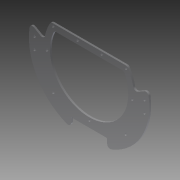
# Autodesk Inventor part: Light Sensor Plate
Saved by Autodesk Inventor 2015 (Build 190159000, 159)
## iProperties
Created: 2016-02-18
Part Number: Light Sensor Plate
Material: Polycarbonate, Clear
Document SubType Name: Modeling
Designer: 23902
Density: 1.2 g/cm^3
Appearance: Polycarbonate - Clear
Mass: 38.1211 g
Surface Area: 243.455 cm^2
Volume: 31.7676 cm^3
Author: 23902
Autodesk Inventor part; units mm, degrees
ref_plane "YZ Plane" through (0, 0, 0) normal (1, 0, 0) x (0, 1, 0)
ref_plane "XZ Plane" through (0, 0, 0) normal (0, 1, 0) x (-1, 0, 0)
ref_plane "XY Plane" through (0, 0, 0) normal (0, 0, 1) x (1, 0, 0)
sketch "Sketch1" plane through (0, 0, 0) normal (0, 1, 0) x (-1, 0, 0)
  circle A0 centre (60.6719, 34.9243) radius 1.6
  circle A1 centre (-60.5717, 34.9243) radius 1.6
  circle A2 centre (0.0501, -70.0757) radius 1.6
  line L0 (-54.4935, 29.9243) -> (54.5936, 29.9243)
  arc A3 (-59.0388, 27.0076) -> (59.1389, 27.0076) centre (0.0501, -0.0757) ccw
  arc A4 (-54.4935, 29.9243) -> (-59.0388, 27.0076) centre (-54.4935, 24.9243) ccw
  arc A5 (59.1389, 27.0076) -> (54.5936, 29.9243) centre (54.5936, 24.9243) ccw
  line L1 (-29.9499, 39.9243) -> (-60.5717, 39.9243)
  line L2 (-29.9499, 39.9243) -> (60.6719, 39.9243)
  arc A6 (-60.5717, 39.9243) -> (-64.9018, 37.4243) centre (-60.5717, 34.9243) ccw
  arc A7 (65.002, 37.4243) -> (60.6719, 39.9243) centre (60.6719, 34.9243) ccw
  line L3 (0.0501, -80.0757) -> (-15.7999, -80.0757)
  line L4 (0.0501, -80.0757) -> (-27.9499, -80.0757)
  arc A8 (-27.9499, -80.0757) -> (-29.9499, -82.0757) centre (-27.9499, -82.0757) ccw
  line L5 (-29.9499, -82.0757) -> (-29.9499, -88.3933)
  arc A9 (-44.5914, -89.5583) -> (-36.792, -93.0416) centre (0.0501, -0.0757) ccw
  arc A10 (-36.792, -93.0416) -> (-29.9499, -88.3933) centre (-34.9499, -88.3933) ccw
  line L6 (0.0501, -80.0757) -> (15.9001, -80.0757)
  line L7 (0.0501, -80.0757) -> (28.0501, -80.0757)
  arc A11 (30.0501, -82.0757) -> (28.0501, -80.0757) centre (28.0501, -82.0757) ccw
  line L8 (30.0501, -82.0757) -> (30.0501, -88.3933)
  arc A12 (36.8922, -93.0416) -> (44.6916, -89.5583) centre (0.0501, -0.0757) ccw
  arc A13 (30.0501, -88.3933) -> (36.8922, -93.0416) centre (35.0501, -88.3933) ccw
  arc A14 (44.6916, -89.5583) -> (98.982, 14.501) centre (0.0501, -0.0757) ccw
  arc A15 (-98.8818, 14.501) -> (-44.5914, -89.5583) centre (0.0501, -0.0757) ccw
  arc A16 (-91.4352, 18.1023) -> (-98.8818, 14.501) centre (-93.9352, 13.7722) ccw
  line L9 (-91.4352, 18.1023) -> (-80.7621, 11.9402)
  arc A17 (-64.9018, 37.4243) -> (-73.3676, 15.2487) centre (0.0501, -0.0757) ccw
  arc A18 (-80.7621, 11.9402) -> (-73.3676, 15.2487) centre (-78.2621, 16.2704) ccw
  arc A19 (98.982, 14.501) -> (91.5354, 18.1023) centre (94.0354, 13.7722) ccw
  line L10 (91.5354, 18.1023) -> (80.8623, 11.9402)
  arc A20 (73.4678, 15.2487) -> (65.002, 37.4243) centre (0.0501, -0.0757) ccw
  arc A21 (73.4678, 15.2487) -> (80.8623, 11.9402) centre (78.3623, 16.2704) ccw
  circle A22 centre (-19.9499, 34.9243) radius 1.6
  circle A23 centre (20.0501, 34.9243) radius 1.6
  circle A24 centre (-60.054, -60.1798) radius 1.6
  circle A25 centre (60.1542, -60.1798) radius 1.6
  circle A26 centre (-91.2981, -14.0713) radius 1.6
  circle A27 centre (-91.2981, 4.9287) radius 1.6
  circle A28 centre (91.3982, -14.0713) radius 1.6
  circle A29 centre (91.3982, 4.9287) radius 1.6
  circle A30 centre (70.8982, -4.5713) radius 1.6
  circle A31 centre (-70.7981, -4.5713) radius 1.6
  constraints: 38 point on circle, 32 centre point, 22 end point, 2 point on line
extrude "Extrusion1" add sketch "Sketch1" along normal blind 3
body "Solid1"
